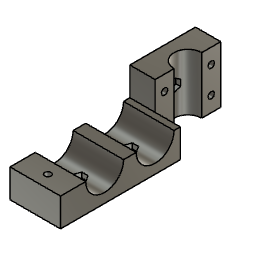
Pressure Clamp v1.0 (Autodesk Fusion 360 design; units mm, degrees)
Autodesk Fusion 360 part; units mm, degrees
sketch "Sketch3" plane through (0, 0, 0) normal (0, 0, 1) x (1, 0, 0)
  circle A0 centre (0, 0) radius 11
  line L0 (0, 11) -> (0, 26)
  line L1 (0, 26) -> (-20, 26)
  line L2 (-20, 26) -> (-20, -26)
  line L3 (-20, -26) -> (0, -26)
  line L4 (0, -26) -> (0, -11)
  line L5 (0, -26) -> (20, -26)
  line L6 (-20, -26) -> (-20, -106)
  line L7 (-20, -106) -> (20, -106)
  line L8 (20, -106) -> (20, -26)
  dimension "d15" = 22
  dimension "d16" = 15
  dimension "d17" = 20
  dimension "d18" = 52
  dimension "d19" = 20
  dimension "d20" = 80
  dimension "d21" = 40
  constraint coincident A0.centre origin
  constraint coincident A0 L0.start
  constraint perpendicular L0 L1
  constraint perpendicular L1 L2
  constraint perpendicular L2 L3
  constraint coincident A0 L4.end
  constraint perpendicular L3 L4
  constraint perpendicular L4 L5
  constraint perpendicular L3 L6
  constraint perpendicular L6 L7
  constraint perpendicular L5 L8
  measures "d15" diameter of A0
  measures "d16" distance of L0.start L0.end
  measures "d17" distance of L0.end L1.end
  measures "d18" distance of L1.end L2.end
  measures "d19" distance of L3.end L5.end
  measures "d20" distance of L2.end L6.end
  measures "d21" distance of L6.end L7.end
extrude "Extrude4" add sketch "Sketch3" along normal blind 45 contours A0 L0 L1 L2 L3 L4
extrude "Extrude5" add sketch "Sketch3" along normal blind 22.5 contours L3 L5 L6 L7 L8
sketch "Sketch4" plane through (-20, 0, 0) normal (-1, 0, 0) x (0, -1, 0)
  line L0 (-26, 0) -> (106, 0)
  line L1 (106, 0) -> (106, 22.5)
  line L2 (106, 22.5) -> (26, 22.5)
  line L3 (26, 22.5) -> (26, 45)
  line L4 (26, 45) -> (-26, 45)
  line L5 (-26, 45) -> (-26, 0)
  line L6 (-26, 45) -> (-18.5, 45) construction
  line L7 (26, 45) -> (18.5, 45) construction
  line L8 (-18.5, 45) -> (-18.5, 33) construction
  circle A0 centre (-18.5, 33) radius 2.5
  circle A1 centre (18.5, 33) radius 2.5
  circle A2 centre (-18.5, 12) radius 2.5
  circle A3 centre (18.5, 12) radius 2.5
  line L9 (-26, 45) -> (26, 45) construction
  line L10 (0, 45) -> (0, 0) construction
  circle A4 centre (0, 22.5) radius 2.5
  dimension "d26" = 7.5
  dimension "d27" = 7.5
  dimension "d28" = 12
  dimension "d29" = 5
  dimension "d32" = 37
  dimension "d33" = -21
  dimension "d36" = 5
  constraint coincident L4.end L5.start
  constraint perpendicular L5 L6
  constraint coincident L3.end L4.start
  constraint perpendicular L3 L7
  constraint perpendicular L0 L8
  constraint coincident L8.end A0.centre
  constraint midpoint L9 L10.start
  constraint coincident L10.end origin
  constraint midpoint L10 A4.centre
  measures "d26" distance of L4.end L6.end
  measures "d27" distance of L3.end L7.end
  measures "d28" distance of L6.end L8.end
  measures "d29" diameter of A0
  measures "d36" diameter of A4
extrude "Extrude6" cut sketch "Sketch4" against normal blind 40 contours A0 | A1 | A2 | A3 | A4
sketch "Sketch5" plane through (-20, 0, 0) normal (-1, 0, 0) x (0, -1, 0)
  circle A0 centre (18.5, 33) radius 2.5
  circle A1 centre (18.5, 12) radius 2.5
  circle A2 centre (-18.5, 33) radius 2.5
  circle A3 centre (-18.5, 12) radius 2.5
  line L0 (-26, 0) -> (106, 0)
  line L1 (106, 0) -> (106, 22.5)
  line L2 (106, 22.5) -> (26, 22.5)
  line L3 (26, 22.5) -> (26, 45)
  line L4 (26, 45) -> (-26, 45)
  line L5 (-26, 45) -> (-26, 0)
  circle A4 centre (0, 22.5) radius 2.5
  circle A5 centre (-18.5, 33) radius 5
  circle A6 centre (18.5, 33) radius 5
  circle A7 centre (-18.5, 12) radius 5
  circle A8 centre (18.5, 12) radius 5
  dimension "d37" = 10
  dimension "d40" = 37
  dimension "d41" = -21
  constraint concentric A2 A5
  measures "d37" diameter of A5
sketch "Sketch6" plane through (-20, 0, 0) normal (-1, 0, 0) x (0, -1, 0)
  line L0 (106, 22.5) -> (86, 22.5) construction
  circle A0 centre (86, 22.5) radius 15
  circle A1 centre (46, 22.5) radius 15
  dimension "d42" = 20
  dimension "d43" = 30
  dimension "d46" = -40
  dimension "d47" = 0
  constraint horizontal L0
  constraint coincident L0.end A0.centre
  measures "d42" distance of L0.start L0.end
  measures "d43" diameter of A0
extrude "Extrude7" cut sketch "Sketch6" against normal blind 400
sketch "Sketch7" plane through (-20, 0, 0) normal (-1, 0, 0) x (0, -1, 0)
  line L0 (0, 22.5) -> (0, 27.5) construction
  line L1 (0, 27.5) -> (-4.3301, 25)
  line L2 (-4.3301, 25) -> (-4.3301, 20)
  line L3 (-4.3301, 20) -> (0, 17.5)
  line L4 (0, 17.5) -> (4.3301, 20)
  line L5 (4.3301, 20) -> (4.3301, 25)
  line L6 (4.3301, 25) -> (0, 27.5)
  point P0 (0, 22.5)
  dimension "d50" = 5
  constraint vertical L0
  constraint coincident P0 L0.start
  constraint coincident L0.end L1.start
  measures "d50" distance of P0 L0.end
extrude "Extrude8" cut sketch "Sketch7" against normal blind 5 from surface at -6
sketch "Sketch8" plane through (0, 0, 0) normal (0, 0, -1) x (1, 0, 0)
  line L0 (0, -26) -> (0, -11)
  arc A0 (0, 11) -> (0, -11) centre (0, 0) ccw
  line L1 (0, 11) -> (0, 26)
  line L2 (0, 26) -> (20, 26)
  line L3 (20, 26) -> (20, 106)
  line L4 (20, 106) -> (-20, 106)
  line L5 (-20, 106) -> (-20, -26)
  line L6 (-20, -26) -> (0, -26)
  line L7 (0, 26) -> (0, 46) construction
  circle A1 centre (0, 46) radius 2.5
  circle A2 centre (0, 86) radius 2.5
  dimension "d54" = 20
  dimension "d55" = 5
  dimension "d58" = 0
  dimension "d59" = 40
  constraint coincident L1.end L2.start
  constraint perpendicular L2 L7
  constraint coincident L7.end A1.centre
  measures "d54" distance of L1.end L7.end
  measures "d55" diameter of A1
extrude "Extrude9" cut sketch "Sketch8" against normal blind 20 contours A1 | A2
sketch "Sketch9" plane through (0, 0, 0) normal (0, 0, -1) x (1, 0, 0)
  circle A0 centre (0, 46) radius 2.5
  circle A1 centre (0, 86) radius 2.5
  line L0 (0, -26) -> (0, -11)
  arc A2 (0, 11) -> (0, -11) centre (0, 0) ccw
  line L1 (0, 11) -> (0, 26)
  line L2 (0, 26) -> (20, 26)
  line L3 (20, 26) -> (20, 106)
  line L4 (20, 106) -> (-20, 106)
  line L5 (-20, 106) -> (-20, -26)
  line L6 (-20, -26) -> (0, -26)
  line L7 (0, 46) -> (-5, 46) construction
  line L8 (0, 86) -> (-5, 86) construction
  line L9 (-5, 46) -> (-2.5, 41.6699)
  line L10 (-2.5, 41.6699) -> (2.5, 41.6699)
  line L11 (2.5, 41.6699) -> (5, 46)
  line L12 (5, 46) -> (2.5, 50.3301)
  line L13 (2.5, 50.3301) -> (-2.5, 50.3301)
  line L14 (-2.5, 50.3301) -> (-5, 46)
  line L15 (-5, 86) -> (-2.5, 81.6699)
  line L16 (-2.5, 81.6699) -> (2.5, 81.6699)
  line L17 (2.5, 81.6699) -> (5, 86)
  line L18 (5, 86) -> (2.5, 90.3301)
  line L19 (2.5, 90.3301) -> (-2.5, 90.3301)
  line L20 (-2.5, 90.3301) -> (-5, 86)
  point P0 (0, 46)
  point P1 (0, 86)
  dimension "d62" = 5
  dimension "d63" = 5
  constraint coincident P0 A0.centre
  constraint horizontal L7
  constraint coincident P1 A1.centre
  constraint horizontal L8
  constraint coincident L7.end L9.start
  constraint coincident L8.end L15.start
  measures "d62" distance of P0 L7.end
  measures "d63" distance of P1 L8.end
extrude "Extrude10" cut sketch "Sketch9" against normal blind 6 from surface at -4 contours L9 L10 L11 L12 L13 L14 | L15 L16 L17 L18 L19 L20
sketch "Sketch10" plane through (-20, 0, 0) normal (-1, 0, 0) x (0, -1, 0)
  arc A0 (71, 22.5) -> (101, 22.5) centre (86, 22.5) ccw
  line L0 (71, 22.5) -> (61, 22.5)
  arc A1 (31, 22.5) -> (61, 22.5) centre (46, 22.5) ccw
  line L1 (31, 22.5) -> (26, 22.5)
  line L2 (26, 22.5) -> (26, 45)
  line L3 (26, 45) -> (-26, 45)
  line L4 (-26, 45) -> (-26, 0)
  line L5 (-26, 0) -> (106, 0)
  line L6 (106, 0) -> (106, 22.5)
  line L7 (106, 22.5) -> (101, 22.5)
  circle A2 centre (0, 22.5) radius 2.5
  circle A3 centre (-18.5, 33) radius 2.5
  circle A4 centre (-18.5, 12) radius 2.5
  circle A5 centre (18.5, 33) radius 2.5
  circle A6 centre (18.5, 12) radius 2.5
  circle A7 centre (-18.5, 12) radius 5
  circle A8 centre (-18.5, 33) radius 5
  circle A9 centre (18.5, 33) radius 5
  circle A10 centre (18.5, 12) radius 5
  dimension "d67" = 10
  dimension "d68" = 10
  dimension "d69" = 10
  dimension "d70" = 10
  constraint concentric A4 A7
  constraint concentric A3 A8
  constraint concentric A5 A9
  constraint concentric A6 A10
  measures "d67" diameter of A7
  measures "d68" diameter of A8
  measures "d69" diameter of A9
  measures "d70" diameter of A10
extrude "Extrude11" cut sketch "Sketch10" against normal blind 5 contours A7 | A8 | A9 | A10
sketch "Sketch11" plane through (0, 0, 0) normal (0, 0, -1) x (1, 0, 0)
  circle A0 centre (0, 46) radius 2.5
  circle A1 centre (0, 86) radius 2.5
  line L0 (0, -26) -> (0, -11)
  arc A2 (0, 11) -> (0, -11) centre (0, 0) ccw
  line L1 (0, 11) -> (0, 26)
  line L2 (0, 26) -> (20, 26)
  line L3 (20, 26) -> (20, 106)
  line L4 (20, 106) -> (-20, 106)
  line L5 (-20, 106) -> (-20, -26)
  line L6 (-20, -26) -> (0, -26)
  line L7 (-20, 106) -> (20, 106)
  line L8 (20, 106) -> (20, 121)
  line L9 (20, 121) -> (-20, 121)
  line L10 (-20, 121) -> (-20, 106)
  dimension "d73" = 15
  constraint horizontal L7
  constraint vertical L8
  constraint horizontal L9
  constraint vertical L10
  constraint coincident L4.end L5.start
  measures "d73" distance of L4.end L9.end
extrude "Extrude12" add sketch "Sketch11" against normal blind 22.5 contours L4 L7 L8 L9 L10
sketch "Sketch12" plane through (0, 0, 22.5) normal (0, 0, 1) x (-1, 0, 0)
  line L0 (-20, 101) -> (20, 101)
  line L1 (20, 101) -> (20, 121)
  line L2 (20, 121) -> (-20, 121)
  line L3 (-20, 121) -> (-20, 101)
  line L4 (0, 101) -> (0, 121) construction
  circle A0 centre (0, 111) radius 2.5
  dimension "d76" = 5
  constraint midpoint L0 L4.start
  constraint midpoint L2 L4.end
  constraint midpoint L4 A0.centre
  measures "d76" diameter of A0
extrude "Extrude13" cut sketch "Sketch12" against normal blind 22.5 contours A0
sketch "Sketch13" plane through (0, 0, 0) normal (0, 0, -1) x (1, 0, 0)
  circle A0 centre (0, 111) radius 2.5
  circle A1 centre (0, 46) radius 2.5
  circle A2 centre (0, 86) radius 2.5
  line L0 (0, -26) -> (0, -11)
  arc A3 (0, 11) -> (0, -11) centre (0, 0) ccw
  line L1 (0, 11) -> (0, 26)
  line L2 (0, 26) -> (20, 26)
  line L3 (20, 26) -> (20, 121)
  line L4 (20, 121) -> (-20, 121)
  line L5 (-20, 121) -> (-20, -26)
  line L6 (-20, -26) -> (0, -26)
  circle A4 centre (0, 111) radius 5
  dimension "d79" = 10
  constraint concentric A0 A4
  measures "d79" diameter of A4
extrude "Extrude14" cut sketch "Sketch13" against normal blind 5 contours A4
equation "d51 = 0 mm - 6.00 mm"
